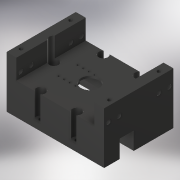
# Autodesk Inventor part: GA01
Saved by Autodesk Inventor 2017 (Build 210142000, 142)
## iProperties
Created: 2018-10-23
Part Number: GA01
Material: ABS Plastic
Document SubType Name: Modeling
Designer: Dell
Density: 1.06 g/cm^3
Appearance: Smooth - Black
Author: Dell
Autodesk Inventor part; units mm, degrees
ref_plane "YZ Plane" through (0, 0, 0) normal (1, 0, 0) x (0, 1, 0)
ref_plane "XZ Plane" through (0, 0, 0) normal (0, 1, 0) x (-1, 0, 0)
ref_plane "XY Plane" through (0, 0, 0) normal (0, 0, 1) x (1, 0, 0)
sketch "Sketch26" plane through (0, 0, 0) normal (0, 0, 1) x (1, 0, 0)
  line L0 (0, 0) -> (140, 0)
  line L1 (140, 0) -> (140, 48)
  line L2 (140, 48) -> (0, 48)
  line L3 (0, 48) -> (0, 0)
  dimension "d137" = 48
  dimension "d138" = 140
  constraints: 8 end point, 2 parallel, 1 horizontal, 1 perpendicular
  measures "d137" distance of L1.end L0.end
  measures "d138" distance of L1.end L2.end
extrude "Extrusion22" add sketch "Sketch26" along normal blind 100
sketch "Sketch27" plane through (0, 48, 0) normal (0, 1, 0) x (1, 0, 0)
  line L0 (0, -100) -> (140, -100) projected
  line L1 (0, 0) -> (140, 0) projected
  line L2 (15, -100) -> (125, -100)
  line L3 (125, -100) -> (125, 0)
  line L4 (125, 0) -> (15, 0)
  line L5 (15, 0) -> (15, -100)
  line L6 (0, 0) -> (0, -100) projected
  line L7 (140, -100) -> (0, -100) projected
  point P0 (70, -100)
  point P1 (70, -100)
  dimension "d141" = 15
  constraints: 8 end point, 4 midpoint, 2 parallel, 2 point on line, 1 horizontal, 1 perpendicular
  measures "d141" distance between parallel lines of L6 L5
extrude "Extrusion23" cut sketch "Sketch27" against normal blind 28 contours L5 L1 L3 L0
sketch "Sketch28" plane through (140, 0, 0) normal (1, 0, 0) x (0, 0, -1)
  circle A0 centre (-93, 28) radius 3
  circle A1 centre (-78, 28) radius 3
  line L0 (-93, 28) -> (-78, 28) construction
  line L1 (0, 48) -> (-100, 48) construction
  line L2 (-50, 48) -> (-50, 0) construction
  line L3 (0, 0) -> (-100, 0) construction
  line L4 (-100, 48) -> (0, 48) construction
  line L5 (-100, 20) -> (-100, 48) construction
  line L6 (-100, 20) -> (0, 20) construction
  line L7 (0, 48) -> (0, 20) construction
  circle A2 centre (-7, 28) radius 3
  circle A3 centre (-22, 28) radius 3
  dimension "d144" = 6
  dimension "d145" = 6
  dimension "d146" = 15
  dimension "d173" = 28
  dimension "d177" = 8
  constraints: 4 centre point, 4 end point, 2 midpoint, 2 symmetric about line, 1 horizontal, 2 other
  measures "d144" diameter of A0
  measures "d145" diameter of A1
  measures "d146" distance of L0.start L0.end
  measures "d173" distance from line of L2 L0.end
  measures "d177" distance from line of L6 L0.start
extrude "Extrusion24" cut sketch "Sketch28" against normal through all
sketch "Sketch30" plane through (0, 0, 0) normal (0, -1, 0) x (1, 0, 0)
  line L0 (63.5, 63.5) -> (39.5, 63.5) construction
  line L1 (39.5, 63.5) -> (39.5, 36.5) construction
  line L2 (39.5, 36.5) -> (63.5, 36.5) construction
  line L3 (63.5, 36.5) -> (63.5, 63.5) construction
  circle A0 centre (70, 50) radius 12.5
  line L4 (140, 0) -> (140, 100) projected
  line L5 (0, 100) -> (140, 100) projected
  circle A1 centre (63.5, 63.5) radius 1.5
  circle A2 centre (63.5, 36.5) radius 1.5
  circle A3 centre (55.5, 63.5) radius 1.5
  circle A4 centre (55.5, 36.5) radius 1.5
  circle A5 centre (47.5, 63.5) radius 1.5
  circle A6 centre (47.5, 36.5) radius 1.5
  circle A7 centre (39.5, 63.5) radius 1.5
  circle A8 centre (39.5, 36.5) radius 1.5
  point P0 (0, 0)
  point P1 (63.5, 50)
  point P2 (140, 50)
  point P3 (70, 100)
  dimension "d153" = 24
  dimension "d154" = 27
  dimension "d155" = 6.5
  dimension "d156" = 25
  dimension "d157" = 3
  dimension "d158" = 3
  dimension "d161" = 8
  constraints: 9 centre point, 8 end point, 3 midpoint, 2 coincident, 2 horizontal, 2 horizontal alignment, 2 parallel, 1 perpendicular, 1 vertical alignment, 12 other
  measures "d153" distance of L2.end L1.end
  measures "d154" distance of L1.end L0.end
  measures "d155" distance from line of L3 A0.centre
  measures "d156" diameter of A0
  measures "d157" diameter of A1
  measures "d158" diameter of A2
  measures "d161" distance of A1.centre A3.centre
extrude "Extrusion26" cut sketch "Sketch30" against normal through all
sketch "Sketch31" plane through (0, 0, 0) normal (0, -1, 0) x (1, 0, 0)
  line L0 (84, 70) -> (29, 70)
  line L1 (29, 70) -> (29, 30)
  line L2 (29, 30) -> (84, 30)
  line L3 (84, 30) -> (84, 70)
  circle A0 centre (70, 50) radius 12.5 projected
  point P0 (0, 0)
  point P1 (84, 50)
  dimension "d168" = 55
  dimension "d169" = 40
  dimension "d170" = 14
  constraints: 8 end point, 2 parallel, 1 horizontal, 1 horizontal alignment, 1 midpoint, 1 perpendicular
  measures "d168" distance of L1.end L2.end
  measures "d169" distance of L2.end L0.start
  measures "d170" distance from line of L3 A0.centre
extrude "Extrusion27" cut sketch "Sketch31" against normal blind 17 contours L3 L2 L1 L0 | A0
sketch "Sketch32" plane through (0, 0, 0) normal (0, -1, 0) x (1, 0, 0)
  line L0 (84, 30) -> (29, 30) projected
  line L1 (29, 30) -> (29, 70) projected
  line L2 (29, 70) -> (84, 70) projected
  line L3 (84, 70) -> (84, 30) projected
  line L4 (84, 30) -> (29, 30) projected
  line L5 (0, 0) -> (140, 0) projected
  line L6 (140, 0) -> (140, 100) projected
  line L7 (0, 100) -> (140, 100) projected
  line L8 (0, 0) -> (0, 100) projected
extrude "Extrusion28" add sketch "Sketch32" along normal blind 25
sketch "Sketch33" plane through (0, 20, 0) normal (0, 1, 0) x (1, 0, 0)
  circle A0 centre (70, -50) radius 12.5 construction
  line L0 (44.5, -94.1673) -> (19, -50) construction
  line L1 (19, -50) -> (44.5, -5.8327) construction
  line L2 (44.5, -5.8327) -> (95.5, -5.8327) construction
  line L3 (95.5, -5.8327) -> (121, -50) construction
  line L4 (121, -50) -> (95.5, -94.1673) construction
  line L5 (95.5, -94.1673) -> (44.5, -94.1673) construction
  circle A1 centre (121, -50) radius 2.5
  circle A2 centre (95.5, -94.1673) radius 2.5
  circle A3 centre (44.5, -94.1673) radius 2.5
  circle A4 centre (19, -50) radius 2.5
  circle A5 centre (44.5, -5.8327) radius 2.5
  circle A6 centre (95.5, -5.8327) radius 2.5
  point P0 (0, 0)
  point P1 (70, -50)
  dimension "d178" = 102
  dimension "d179" = 5
  dimension "d180" = 5
  dimension "d181" = 5
  dimension "d182" = 5
  dimension "d183" = 5
  dimension "d184" = 5
  constraints: 12 end point, 7 coincident, 6 centre point, 1 horizontal, 13 other
  measures "d178" distance of L0.end L3.end
  measures "d179" diameter of A1
  measures "d180" diameter of A2
  measures "d181" diameter of A3
  measures "d182" diameter of A4
  measures "d183" diameter of A5
  measures "d184" diameter of A6
extrude "Extrusion29" cut sketch "Sketch33" against normal through all
sketch "Sketch34" plane through (0, 20, 0) normal (0, 1, 0) x (1, 0, 0)
  circle A0 centre (70, -50) radius 12.5 projected
  circle A1 centre (95.5, -5.8327) radius 2.5 projected
  circle A2 centre (95.5, -5.8327) radius 6.5
  circle A3 centre (44.5, -5.8327) radius 6.5
  circle A4 centre (19, -50) radius 6.5
  circle A5 centre (44.5, -94.1673) radius 6.5
  circle A6 centre (95.5, -94.1673) radius 6.5
  circle A7 centre (121, -50) radius 6.5
  point P0 (0, 0)
  dimension "d187" = 13
  dimension "d190" = 360
  constraints: 6 centre point, 1 coincident, 13 other
  measures "d187" diameter of A2
extrude "Extrusion30" cut sketch "Sketch34" along normal blind 50 and the other way blind 35 contours A0 | A1 | A2 | A3 | A4 | A5 | A6 | A7
sketch "Sketch35" plane through (0, -25, 0) normal (0, -1, 0) x (1, 0, 0)
  circle A0 centre (44.5, 5.8327) radius 2.5 construction
  circle A1 centre (44.5, 94.1673) radius 2.5 construction
  circle A2 centre (121, 50) radius 2.5 construction
  circle A3 centre (95.5, 94.1673) radius 2.5 construction
  circle A4 centre (19, 50) radius 2.5 construction
  circle A5 centre (95.5, 5.8327) radius 2.5 construction
  line L0 (29, 70) -> (84, 70) projected
  line L1 (84, 70) -> (84, 30) projected
  line L2 (84, 30) -> (29, 30) projected
  line L3 (29, 30) -> (29, 70) projected
  line L4 (0, 0) -> (140, 0) construction
  line L5 (140, 0) -> (140, 100) construction
  line L6 (140, 100) -> (0, 100) construction
  line L7 (0, 100) -> (0, 0) construction
  line L8 (84, 30) -> (111, 30)
  line L9 (111, 30) -> (111, 70)
  line L10 (111, 70) -> (84, 70)
  line L11 (84, 70) -> (84, 30)
  dimension "d196" = 27
  constraints: 8 end point, 2 parallel, 1 horizontal, 1 horizontal alignment, 1 perpendicular
  measures "d196" distance of L1.end L8.end
extrude "Extrusion31" cut sketch "Sketch35" against normal blind 25 contours L10 L9 L8 L1
sketch "Sketch36" plane through (140, 48, 100) normal (0, 1, 0) x (1, 0, 0)
  line L0 (-7.5, 15) -> (-7.5, 85) construction
  circle A0 centre (-7.5, 15) radius 2.5
  circle A1 centre (-7.5, 85) radius 2.5
  line L1 (0, 0) -> (-15, 0) construction
  line L2 (0, 100) -> (0, 0) construction
  circle A2 centre (-70, 50) radius 12.5 construction
  line L3 (-70, 50) -> (-70, 0) construction
  line L4 (-47.3687, 0) -> (-92.6313, 0) construction
  circle A3 centre (-132.5, 15) radius 2.5
  circle A4 centre (-132.5, 85) radius 2.5
  point P0 (-7.5, 50)
  point P1 (-7.5, 0)
  point P2 (0, 50)
  dimension "d199" = 5
  dimension "d200" = 5
  dimension "d201" = 70
  constraints: 4 centre point, 4 end point, 4 midpoint, 2 coincident, 2 symmetric about line, 2 vertical, 1 horizontal alignment, 1 vertical alignment, 2 other
  measures "d199" diameter of A0
  measures "d200" diameter of A1
  measures "d201" distance of L0.start L0.end
extrude "Extrusion32" cut sketch "Sketch36" against normal through all
sketch "Sketch37" plane through (0, 0, 0) normal (0, -1, 0) x (1, 0, 0)
  line L0 (84, 62.0836) -> (140, 62.0836)
  line L1 (140, 62.0836) -> (140, 82.0836)
  line L2 (140, 82.0836) -> (84, 82.0836)
  line L3 (84, 82.0836) -> (84, 62.0836)
  arc A0 (92.6313, 100) -> (98.3687, 100) centre (95.5, 94.1673) ccw construction
  arc A1 (125, 55.1235) -> (125, 44.8765) centre (121, 50) ccw construction
  line L4 (95.5, 94.1673) -> (121, 94.1673) construction
  line L5 (121, 94.1673) -> (121, 50) construction
  line L6 (84, 70) -> (84, 30) projected
  line L7 (140, 0) -> (140, 100) projected
  point P0 (0, 0)
  point P1 (84, 72.0836)
  point P2 (121, 72.0836)
  dimension "d204" = 20
  constraints: 12 end point, 2 horizontal, 2 midpoint, 2 parallel, 2 perpendicular, 2 point on line, 1 horizontal alignment
  measures "d204" distance of L0.end L1.end
extrude "Extrusion33" cut sketch "Sketch37" along normal blind 20
sketch "Sketch38" plane through (0, 48, 100) normal (0, 1, 0) x (1, 0, 0)
  line L0 (15, 0) -> (0, 0) projected
  line L1 (140, 100) -> (125, 100) projected
  line L2 (0, 100) -> (0, 0) projected
  line L3 (140, 100) -> (140, 0) projected
  line L4 (0, 0) -> (140, 0)
  line L5 (140, 0) -> (140, 100)
  line L6 (140, 100) -> (0, 100)
  line L7 (0, 100) -> (0, 0)
  line L8 (139, 1) -> (1, 1)
  line L9 (1, 1) -> (1, 99)
  line L10 (1, 99) -> (139, 99)
  line L11 (139, 99) -> (139, 1)
  dimension "d207" = 1
  constraints: 16 end point, 4 parallel, 2 perpendicular, 1 horizontal, 3 other
  measures "d207" distance between parallel lines of L4 L8
extrude "Extrusion34" cut sketch "Sketch38" against normal through all
sketch "Sketch39" plane through (0, 0, 0) normal (0, -1, 0) x (1, 0, 0)
  line L0 (139, 62.0836) -> (139, 82.0836) projected
  line L1 (139, 82.0836) -> (84, 82.0836) projected
  line L2 (84, 82.0836) -> (84, 70) projected
  line L3 (84, 30) -> (84, 70) projected
  line L4 (111, 30) -> (84, 30) projected
  line L5 (111, 62.0836) -> (111, 30) projected
  line L6 (111, 62.0836) -> (139, 62.0836) projected
  arc A0 (48.8468, 1) -> (40.1532, 1) centre (44.5, 5.8327) ccw projected
  arc A1 (99.8468, 1) -> (91.1532, 1) centre (95.5, 5.8327) ccw projected
  arc A2 (40.1532, 99) -> (48.8468, 99) centre (44.5, 94.1673) ccw projected
  circle A3 centre (19, 50) radius 6.5 projected
  arc A4 (91.1532, 99) -> (99.8468, 99) centre (95.5, 94.1673) ccw projected
  circle A5 centre (121, 50) radius 6.5 projected
  line L7 (127.5, 82.0836) -> (19, 82.0836)
  line L8 (19, 82.0836) -> (19, 86.1673)
  line L9 (19, 86.1673) -> (127.5, 86.1673)
  line L10 (127.5, 86.1673) -> (127.5, 82.0836)
  line L11 (29, 70) -> (84, 70) projected
  line L12 (84, 70) -> (19, 70)
  line L13 (19, 70) -> (19, 82.0836)
  line L14 (19, 82.0836) -> (84, 82.0836)
  line L15 (84, 82.0836) -> (84, 70)
  line L16 (111, 42) -> (127.5, 42)
  line L17 (127.5, 42) -> (127.5, 13.8327)
  line L18 (127.5, 13.8327) -> (111, 13.8327)
  line L19 (111, 13.8327) -> (111, 42)
  line L20 (127.5, 13.8327) -> (19, 13.8327)
  line L21 (19, 13.8327) -> (19, 30)
  line L22 (19, 30) -> (127.5, 30)
  line L23 (127.5, 30) -> (127.5, 13.8327)
  circle A6 centre (132.5, 85) radius 2.5 projected
  point P0 (0, 0)
  point P1 (29, 30)
  dimension "d210" = 5
  dimension "d211" = 8
  dimension "d212" = 8
  dimension "d213" = 8
  constraints: 32 end point, 8 parallel, 4 horizontal, 4 perpendicular, 3 point on line, 3 vertical alignment
  measures "d210" distance from line of L10 A6.centre
  measures "d211" distance from line of A0.centre L20
  measures "d212" distance from line of L16 A5.centre
  measures "d213" distance from line of A2.centre L9
extrude "Extrusion35" cut sketch "Sketch39" along normal through all contours L6 L5 L4 L3 L2 L1 L0 | L1 L7 L8 L9 L10 | L2 L11 L12 L13 L7 | L19 L20 L21 L22 L4 | L22 L17 L18 L19
sketch "Sketch41" plane through (1, 48, 1) normal (-1, 0, 0) x (0, 0, 1)
  line L0 (69, -48) -> (69, -73) projected
  line L1 (69, -48) -> (69, -73) projected
  line L2 (29, -73) -> (29, -48) projected
  line L3 (29, -48) -> (29, -73) projected
  line L4 (29, -73) -> (29, -48) projected
  line L5 (29, -48) -> (69, -48)
  line L6 (69, -48) -> (69, -73)
  line L7 (69, -73) -> (29, -73)
  line L8 (29, -73) -> (29, -48)
  line L9 (29, -48) -> (19, -48)
  line L10 (19, -48) -> (19, -73)
  line L11 (19, -73) -> (29, -73)
  line L12 (29, -73) -> (29, -48)
  point P0 (-1, -48)
  dimension "d218" = 10
  constraints: 16 end point, 4 parallel, 2 horizontal, 2 perpendicular, 1 horizontal alignment
  measures "d218" distance between parallel lines of L10 L2
extrude "Extrusion36" cut sketch "Sketch41" against normal blind 5 contours L0 L7 L2 L5
extrude "Extrusion37" cut sketch "Sketch41" against normal blind 20 contours L2 L11 L10 L9
sketch "Sketch42" plane through (0, 0, 0) normal (0, -1, 0) x (1, 0, 0)
  line L0 (29, 70) -> (84, 70) projected
  line L1 (19, 86.1673) -> (19, 70) projected
  line L2 (29, 70) -> (19, 70)
  line L3 (19, 70) -> (19, 86.1673)
  line L4 (19, 86.1673) -> (29, 86.1673)
  line L5 (29, 86.1673) -> (29, 70)
  point P0 (0, 0)
  constraints: 8 end point, 2 parallel, 1 horizontal, 1 perpendicular
extrude "Extrusion38" add sketch "Sketch42" along normal blind 25
sketch "Sketch43" plane through (0, 0, 0) normal (0, -1, 0) x (1, 0, 0)
  line L0 (111, 62.0836) -> (111, 30) projected
  line L1 (127.5, 13.8327) -> (19, 13.8327) projected
  line L2 (111, 30) -> (127.5, 30)
  line L3 (127.5, 30) -> (127.5, 13.8327)
  line L4 (127.5, 13.8327) -> (111, 13.8327)
  line L5 (111, 13.8327) -> (111, 30)
  point P0 (0, 0)
  constraints: 8 end point, 2 parallel, 1 horizontal, 1 perpendicular
extrude "Extrusion39" add sketch "Sketch43" along normal blind 25
sketch "Sketch44" plane through (0, 0, 0) normal (0, -1, 0) x (1, 0, 0)
  line L0 (139, 62.0836) -> (111, 62.0836) projected
  line L1 (111, 62.0836) -> (111, 13.8327) projected
  line L2 (139, 62.0836) -> (111, 62.0836)
  line L3 (111, 62.0836) -> (111, 57.0836)
  line L4 (111, 57.0836) -> (139, 57.0836)
  line L5 (139, 57.0836) -> (139, 62.0836)
  point P0 (0, 0)
  dimension "d225" = 5
  constraints: 8 end point, 2 parallel, 1 horizontal, 1 perpendicular, 1 point on line
  measures "d225" distance between parallel lines of L4 L0
extrude "Extrusion40" cut sketch "Sketch44" along normal through all
sketch "Sketch45" plane through (0, 0, 0) normal (0, -1, 0) x (1, 0, 0)
  line L0 (127.5, 82.0836) -> (139, 82.0836) projected
  line L1 (139, 82.0836) -> (139, 57.0836) projected
  line L2 (127.5, 82.0836) -> (139, 82.0836)
  line L3 (139, 82.0836) -> (139, 77.0836)
  line L4 (139, 77.0836) -> (127.5, 77.0836)
  line L5 (127.5, 77.0836) -> (127.5, 82.0836)
  point P0 (0, 0)
  dimension "d228" = 5
  constraints: 8 end point, 2 parallel, 1 horizontal, 1 perpendicular, 1 point on line
  measures "d228" distance between parallel lines of L0 L4
extrude "Extrusion41" add sketch "Sketch45" along normal blind 25
sketch "Sketch46" plane through (0, 0, 0) normal (0, -1, 0) x (1, 0, 0)
  line L0 (127.5, 77.0836) -> (139, 77.0836) projected
  line L1 (29, 86.1673) -> (127.5, 86.1673) projected
  line L2 (127.5, 77.0836) -> (29, 77.0836)
  line L3 (29, 77.0836) -> (29, 86.1673)
  line L4 (29, 86.1673) -> (127.5, 86.1673)
  line L5 (127.5, 86.1673) -> (127.5, 77.0836)
  point P0 (0, 0)
  constraints: 8 end point, 2 parallel, 1 horizontal, 1 perpendicular
extrude "Extrusion42" add sketch "Sketch46" along normal blind 25
sketch "Sketch47" plane through (0, 0, 0) normal (0, -1, 0) x (1, 0, 0)
  line L0 (29, 30) -> (29, 70) projected
  line L1 (29, 77.0836) -> (139, 77.0836) projected
  line L2 (29, 70) -> (84, 70)
  line L3 (84, 70) -> (84, 77.0836)
  line L4 (84, 77.0836) -> (29, 77.0836)
  line L5 (29, 77.0836) -> (29, 70)
  point P0 (0, 0)
  constraints: 8 end point, 2 parallel, 1 horizontal, 1 midpoint, 1 perpendicular
extrude "Extrusion43" add sketch "Sketch47" along normal blind 25
sketch "Sketch48" plane through (0, 0, 0) normal (0, -1, 0) x (1, 0, 0)
  line L0 (84, 77.0836) -> (84, 70) construction
  line L1 (84, 30) -> (84, 70) construction
  line L2 (29, 30) -> (84, 30) construction
  line L3 (29, 30) -> (6, 30) construction
  line L4 (6, 30) -> (6, 70) construction
  line L5 (1, 70) -> (6, 70) construction
  line L6 (1, 20) -> (1, 70) construction
  line L7 (1, 20) -> (19, 20) construction
  line L8 (19, 20) -> (19, 13.8327) construction
  line L9 (19, 13.8327) -> (111, 13.8327) construction
  line L10 (111, 13.8327) -> (111, 57.0836) construction
  line L11 (111, 57.0836) -> (139, 57.0836) construction
  line L12 (139, 77.0836) -> (139, 57.0836) construction
  line L13 (139, 77.0836) -> (84, 77.0836) construction
  circle A0 centre (97.5, 25.4582) radius 1.5
  circle A1 centre (97.5, 45.4582) radius 1.5
  line L14 (111, 57.0836) -> (84, 57.0836) construction
  line L15 (84, 70) -> (84, 30) construction
  line L16 (97.5, 25.4582) -> (97.5, 45.4582) construction
  point P0 (0, 0)
  point P1 (97.5, 57.0836)
  point P2 (97.5, 35.4582)
  point P3 (111, 35.4582)
  dimension "d235" = 3
  dimension "d236" = 3
  dimension "d237" = 20
  constraints: 4 end point, 3 midpoint, 2 centre point, 1 horizontal alignment, 1 perpendicular, 1 point on line, 1 vertical, 1 vertical alignment
  measures "d235" diameter of A0
  measures "d236" diameter of A1
  measures "d237" distance of L16.start L16.end
extrude "Extrusion44" cut sketch "Sketch48" against normal blind 12
sketch "Sketch49" plane through (6, 48, 1) normal (-1, 0, 0) x (0, 0, 1)
  line L0 (69, -48) -> (69, -73) projected
  line L1 (29, -48) -> (69, -48) projected
  line L2 (29, -73) -> (29, -48) projected
  line L3 (69, -73) -> (29, -73) projected
  circle A0 centre (34, -53) radius 1.5
  circle A1 centre (64, -68) radius 1.5
  point P0 (-1, -48)
  dimension "d240" = 3
  dimension "d241" = 3
  dimension "d242" = 5
  dimension "d243" = 5
  dimension "d244" = 5
  dimension "d245" = 5
  constraints: 2 centre point
  measures "d240" diameter of A0
  measures "d241" diameter of A1
  measures "d242" distance from line of L2 A0.centre
  measures "d243" distance from line of L1 A0.centre
  measures "d244" distance from line of L0 A1.centre
  measures "d245" distance from line of L3 A1.centre
extrude "Extrusion45" cut sketch "Sketch49" against normal blind 25 contours A0 | A1
sketch "Sketch50" plane through (1, 48, 1) normal (-1, 0, 0) x (0, 0, 1)
  circle A0 centre (91, -60.5) radius 1.5
  circle A1 centre (7, -60.5) radius 1.5
  line L0 (69, -48) -> (69, -73) projected
  line L1 (0, 0) -> (0, -73) projected
  line L2 (98, 0) -> (98, -73) projected
  point P0 (-1, -48)
  point P1 (69, -60.5)
  point P2 (69, -60.5)
  dimension "d248" = 3
  dimension "d249" = 3
  dimension "d250" = 7
  dimension "d251" = 7
  constraints: 2 centre point, 2 horizontal alignment, 2 midpoint
  measures "d248" diameter of A0
  measures "d249" diameter of A1
  measures "d250" distance from line of L1 A1.centre
  measures "d251" distance from line of L2 A0.centre
extrude "Extrusion46" cut sketch "Sketch50" against normal blind 12
body "Solid2"
